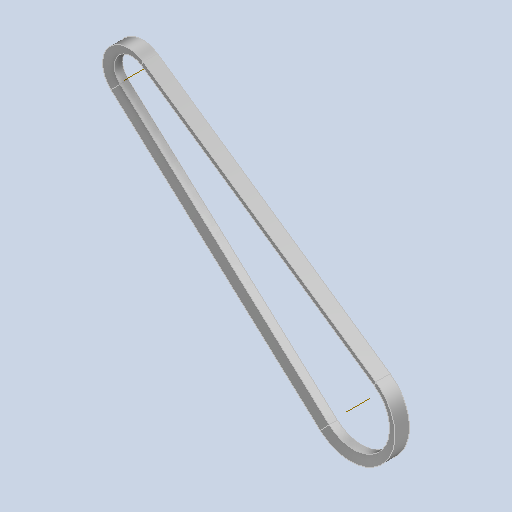
# Autodesk Inventor part: Клиновой ремень
Saved by Autodesk Inventor 2023 (Build 270158000, 158)
## iProperties
Created: 2022-05-23
Part Number: Клиновой ремень
Material: Rubber
Document SubType Name: Modeling
Designer: avkap
Density: 0.93 g/cm^3
Appearance: Rubber - Black - Version 1.1
CustomPartVersion: 1
Author: avkap
Autodesk Inventor part; units mm, degrees
ref_plane "YZ Plane" through (0, 0, 0) normal (1, 0, 0) x (0, 1, 0)
ref_plane "XZ Plane" through (0, 0, 0) normal (0, 1, 0) x (-1, 0, 0)
sketch "Эскизная траектория" plane through (0, 0, 0) normal (0, 0, 1) x (1, 0, 0)
  arc A0 (23.7284, 6.4029) -> (-2.0695, -26.0498) centre (11.9109, -10.6831) ccw
  arc A1 (192.1481, -202.7473) -> (239.6775, -142.9574) centre (217.9052, -174.4363) ccw
  line L0 (192.1481, -202.7473) -> (-2.0695, -26.0498)
  line L1 (23.7284, 6.4029) -> (239.6775, -142.9574)
  constraints: 4 end point, 4 point on circle, 2 centre point
ref_plane "Плоскость сечения" through (-2.0695, -26.0498, 0) normal (0.7397, -0.673, 0) x (0, 0, 1)
sketch "Сечение" plane through (-2.0695, -26.0498, 0) normal (0.7397, -0.673, 0) x (0, 0, 1)
  line L0 (0, 3.2254) -> (0, -4.7746) construction
  line L1 (-5.5, 0) -> (5.5, 0) construction
  line L2 (-6.6739, 3.2254) -> (6.6739, 3.2254)
  line L3 (6.6739, 3.2254) -> (3.7622, -4.7746)
  line L4 (3.7622, -4.7746) -> (-3.7622, -4.7746)
  line L5 (-3.7622, -4.7746) -> (-6.6739, 3.2254)
  point P0 (0, 0)
  point P1 (0, 0)
  point P2 (0, 0)
  dimension "d0" = 11
  dimension "d1" = 3.2254
  dimension "d2" = 40
  dimension "d3" = 8
  constraints: 12 end point, 3 midpoint, 2 parallel, 2 point on line, 1 coincident, 1 perpendicular, 1 vertical, 1 other
  measures "d0" distance of L1.start L1.end
  measures "d1" distance between parallel lines of L2 L1
  measures "d2" angle of L5 L3
  measures "d3" distance between parallel lines of L4 L2
sweep "Ремень" add profiles "Сечение" path "Эскизная траектория"
equation "\"d0\" = da_Bw"
equation "\"d1\" = da_Hw"
equation "\"d2\" = da_Alfa"
equation "\"d3\" = da_H"
equation "\"da_Alfa\" = 40deg"
equation "\"da_H\" = 8"
equation "\"da_Bw\" = 11"
equation "\"da_Hw\" = 3.22535"
body "Solid1"
